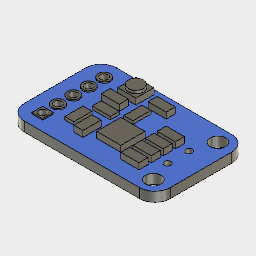
2130 PAM8302 (Autodesk Fusion 360 design; units mm, degrees)
Autodesk Fusion 360 part; units mm, degrees
sketch "Sketch1" plane through (0, 0, 0) normal (0, 0, 1) x (1, 0, 0)
  arc A0 (21.59, 0) -> (24.13, 2.54) centre (21.59, 2.54) ccw
  arc A1 (0, 2.54) -> (2.54, 0) centre (2.54, 2.54) ccw
  line L0 (21.59, 0) -> (2.54, 0)
  arc A2 (2.54, 15.24) -> (0, 12.7) centre (2.54, 12.7) ccw
  line L1 (24.13, 12.7) -> (24.13, 2.54)
  line L2 (0, 2.54) -> (0, 12.7)
  line L3 (2.54, 15.24) -> (21.59, 15.24)
  arc A3 (24.13, 12.7) -> (21.59, 15.24) centre (21.59, 12.7) ccw
  arc A4 (20.9931, 9.293) -> (19.9009, 9.293) centre (20.447, 9.293) ccw
  line L4 (2.159, 1.651) -> (3.937, 1.651)
  line L5 (3.937, 1.651) -> (3.937, 3.429)
  line L6 (2.159, 1.651) -> (3.937, 1.651)
  line L7 (3.937, 1.651) -> (3.937, 3.429)
  line L8 (3.937, 3.429) -> (2.159, 3.429)
  arc A5 (20.9931, 5.793) -> (19.9009, 5.793) centre (20.447, 5.793) ccw
  arc A6 (19.9009, 9.293) -> (20.9931, 9.293) centre (20.447, 9.293) ccw
  arc A7 (19.9009, 9.293) -> (20.9931, 9.293) centre (20.447, 9.293) ccw
  line L9 (2.159, 3.429) -> (2.159, 1.651)
  line L10 (2.159, 3.429) -> (2.159, 1.651)
  arc A8 (20.9931, 9.293) -> (19.9009, 9.293) centre (20.447, 9.293) ccw
  arc A9 (19.9009, 5.793) -> (20.9931, 5.793) centre (20.447, 5.793) ccw
  arc A10 (20.9931, 5.793) -> (19.9009, 5.793) centre (20.447, 5.793) ccw
  line L11 (3.937, 3.429) -> (2.159, 3.429)
  arc A11 (19.9009, 5.793) -> (20.9931, 5.793) centre (20.447, 5.793) ccw
  circle A12 centre (21.59, 2.286) radius 1.27
  circle A13 centre (21.59, 12.954) radius 1.27
  circle A14 centre (3.048, 2.54) radius 0.635
  circle A15 centre (3.048, 5.08) radius 0.635
  circle A16 centre (3.048, 7.62) radius 0.635
  circle A17 centre (3.048, 10.16) radius 0.635
  circle A18 centre (3.048, 12.7) radius 0.635
  circle A19 centre (3.048, 5.08) radius 1
  circle A20 centre (3.048, 7.62) radius 1
  circle A21 centre (3.048, 10.16) radius 1
  circle A22 centre (3.048, 12.7) radius 1
  dimension "d1" = 2.54
  dimension "d2" = 2.54
  dimension "d5" = 1.27
  dimension "d8" = 0
  dimension "d9" = 2.54
  dimension "d10" = 2
  dimension "d13" = 0
  dimension "d14" = 2.54
  measures "d1" diameter of A12
  measures "d2" diameter of A13
  measures "d5" diameter of A14
  measures "d10" diameter of A19
extrude "Extrude1" add sketch "Sketch1" along normal blind 1.6 contours A0 A1 L0 A2 L1 L2 L3 A3 | L4 L5 L6 L7 L8 L9 L10 L11 | A19 | A20 | A21 | A22
extrude "Extrude2" add sketch "Sketch1" along normal blind 0.2 from surface at 1.6 contours L4 L5 L6 L7 L8 L9 L10 L11 | A19 | A20 | A21 | A22
sketch "Sketch2" plane through (0, 0, 1.6) normal (0, 0, 1) x (-1, 0, 0)
  circle A0 centre (-3.048, -12.7) radius 1
  line L0 (-3.937, -1.651) -> (-2.159, -1.651)
  line L1 (-2.159, -1.651) -> (-2.159, -3.429)
  line L2 (-2.159, -3.429) -> (-3.937, -3.429)
  line L3 (-3.937, -3.429) -> (-3.937, -1.651)
  circle A1 centre (-3.048, -10.16) radius 1
  circle A2 centre (-3.048, -5.08) radius 1
  circle A3 centre (-3.048, -7.62) radius 1
  circle A4 centre (-21.59, -2.286) radius 1.27
  circle A5 centre (-20.447, -9.293) radius 0.5461
  circle A6 centre (-21.59, -12.954) radius 1.27
  circle A7 centre (-20.447, -5.793) radius 0.5461
  arc A8 (-21.59, 0) -> (-24.13, -2.54) centre (-21.59, -2.54) ccw
  line L4 (-24.13, -2.54) -> (-24.13, -12.7)
  arc A9 (-24.13, -12.7) -> (-21.59, -15.24) centre (-21.59, -12.7) ccw
  line L5 (-21.59, -15.24) -> (-2.54, -15.24)
  arc A10 (-2.54, -15.24) -> (0, -12.7) centre (-2.54, -12.7) ccw
  line L6 (0, -12.7) -> (0, -2.54)
  arc A11 (0, -2.54) -> (-2.54, 0) centre (-2.54, -2.54) ccw
  line L7 (-2.54, 0) -> (-21.59, 0)
  line L8 (-7.25, -3.5) -> (-5.75, -3.5)
  line L9 (-5.75, -3.5) -> (-5.75, -6.5)
  line L10 (-5.75, -6.5) -> (-7.25, -6.5)
  line L11 (-7.25, -6.5) -> (-7.25, -3.5)
  line L12 (-7.25, -3.5) -> (-5.75, -6.5) construction
  line L13 (-5.75, -3.5) -> (-7.25, -6.5) construction
  line L14 (-9.75, -2.5) -> (-8.25, -2.5)
  line L15 (-8.25, -2.5) -> (-8.25, -5.5)
  line L16 (-8.25, -5.5) -> (-9.75, -5.5)
  line L17 (-9.75, -5.5) -> (-9.75, -2.5)
  line L18 (-9.75, -2.5) -> (-8.25, -5.5) construction
  line L19 (-8.25, -2.5) -> (-9.75, -5.5) construction
  line L20 (-15, -3.5) -> (-11, -3.5)
  line L21 (-11, -3.5) -> (-11, -7.5)
  line L22 (-11, -7.5) -> (-15, -7.5)
  line L23 (-15, -7.5) -> (-15, -3.5)
  line L24 (-15, -3.5) -> (-11, -7.5) construction
  line L25 (-11, -3.5) -> (-15, -7.5) construction
  line L26 (-9, -9.25) -> (-6, -9.25)
  line L27 (-6, -9.25) -> (-6, -10.75)
  line L28 (-6, -10.75) -> (-9, -10.75)
  line L29 (-9, -10.75) -> (-9, -9.25)
  line L30 (-9, -9.25) -> (-6, -10.75) construction
  line L31 (-6, -9.25) -> (-9, -10.75) construction
  line L32 (-6.5, -7.25) -> (-9.5, -7.25)
  line L33 (-9.5, -7.25) -> (-9.5, -8.75)
  line L34 (-9.5, -8.75) -> (-6.5, -8.75)
  line L35 (-6.5, -8.75) -> (-6.5, -7.25)
  line L36 (-6.5, -7.25) -> (-9.5, -8.75) construction
  line L37 (-9.5, -7.25) -> (-6.5, -8.75) construction
  circle A12 centre (-8, -13) radius 1.25
  line L38 (-14, -12) -> (-11, -12)
  line L39 (-11, -12) -> (-11, -13.5)
  line L40 (-11, -13.5) -> (-14, -13.5)
  line L41 (-14, -13.5) -> (-14, -12)
  line L42 (-14, -12) -> (-11, -13.5) construction
  line L43 (-11, -12) -> (-14, -13.5) construction
  line L44 (-12, -8.5) -> (-10.5, -8.5)
  line L45 (-10.5, -8.5) -> (-10.5, -11.5)
  line L46 (-10.5, -11.5) -> (-12, -11.5)
  line L47 (-12, -11.5) -> (-12, -8.5)
  line L48 (-12, -8.5) -> (-10.5, -11.5) construction
  line L49 (-10.5, -8.5) -> (-12, -11.5) construction
  line L50 (-19, -2.5) -> (-16, -2.5)
  line L51 (-16, -2.5) -> (-16, -4)
  line L52 (-16, -4) -> (-19, -4)
  line L53 (-19, -4) -> (-19, -2.5)
  line L54 (-19, -2.5) -> (-16, -4) construction
  line L55 (-16, -2.5) -> (-19, -4) construction
  line L56 (-19, -6) -> (-19, -4.5)
  line L57 (-19, -4.5) -> (-16, -4.5)
  line L58 (-16, -4.5) -> (-16, -6)
  line L59 (-16, -6) -> (-19, -6)
  line L60 (-19, -8) -> (-19, -6.5)
  line L61 (-19, -6.5) -> (-16, -6.5)
  line L62 (-16, -6.5) -> (-16, -8)
  line L63 (-16, -8) -> (-19, -8)
  line L64 (-19, -10) -> (-19, -8.5)
  line L65 (-19, -8.5) -> (-16, -8.5)
  line L66 (-16, -8.5) -> (-16, -10)
  line L67 (-16, -10) -> (-19, -10)
  line L68 (-6.5, -11.5) -> (-9.5, -11.5)
  line L69 (-9.5, -11.5) -> (-9.5, -14.5)
  line L70 (-9.5, -14.5) -> (-6.5, -14.5)
  line L71 (-6.5, -14.5) -> (-6.5, -11.5)
  line L72 (-6.5, -11.5) -> (-9.5, -14.5) construction
  line L73 (-9.5, -11.5) -> (-6.5, -14.5) construction
  point P0 (-6.5, -5)
  point P1 (-9, -4)
  point P2 (-13, -5.5)
  point P3 (-7.5, -10)
  point P4 (-8, -8)
  point P5 (-12.5, -12.75)
  point P6 (-11.25, -10)
  point P7 (-17.5, -3.25)
  point P8 (-8, -13)
  dimension "d18" = 1.5
  dimension "d19" = 3
  dimension "d20" = 1.5
  dimension "d21" = 3
  dimension "d22" = 4
  dimension "d23" = 4
  dimension "d24" = 3
  dimension "d25" = 1.5
  dimension "d26" = 3
  dimension "d27" = 1.5
  dimension "d28" = 2.5
  dimension "d29" = 1.5
  dimension "d30" = 3
  dimension "d31" = 3
  dimension "d32" = 1.5
  dimension "d33" = 3
  dimension "d34" = 1.5
  dimension "d37" = 0
  dimension "d38" = -2
  dimension "d43" = 3
  dimension "d44" = 3
  measures "d18" distance of L9.end L10.end
  measures "d19" distance of L14.end L15.end
  measures "d20" distance of L15.end L16.end
  measures "d21" distance of L8.end L9.end
  measures "d22" distance of L21.end L22.end
  measures "d23" distance of L20.end L21.end
  measures "d24" distance of L27.end L28.end
  measures "d25" distance of L26.end L27.end
  measures "d26" distance of L33.end L34.end
  measures "d27" distance of L32.end L33.end
  measures "d28" diameter of A12
  measures "d29" distance of L38.end L39.end
  measures "d30" distance of L39.end L40.end
  measures "d31" distance of L44.end L45.end
  measures "d32" distance of L45.end L46.end
  measures "d33" distance of L51.end L52.end
  measures "d34" distance of L50.end L51.end
  measures "d43" distance of L69.end L70.end
  measures "d44" distance of L68.end L69.end
extrude "Extrude3" add sketch "Sketch2" along normal blind 0.5 contours L8 L9 L10 L11 | L32 L33 L34 L35 | L44 L45 L46 L47
extrude "Extrude4" add sketch "Sketch2" along normal blind 1 contours L14 L15 L16 L17 | L20 L21 L22 L23 | L26 L27 L28 L29 | L38 L39 L40 L41 | L50 L51 L52 L53 | L56 L57 L58 L59 | L60 L61 L62 L63 | L64 L65 L66 L67
extrude "Extrude5" add sketch "Sketch2" along normal blind 1 contours A12 | L68 L69 L70 L71
extrude "Extrude6" add sketch "Sketch2" along normal blind 0.5 from surface at 1 contours A12
